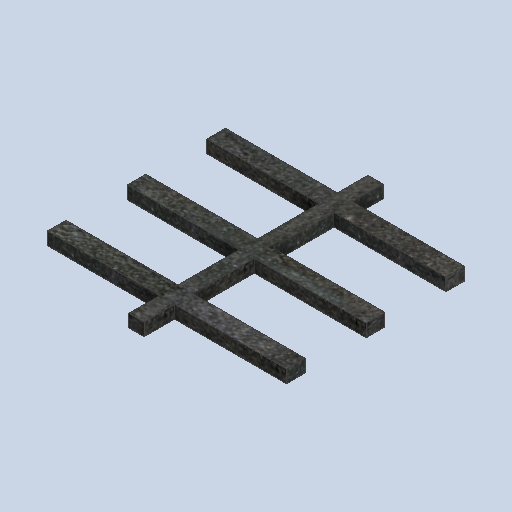
# Autodesk Inventor part: Grid RS3
Saved by Autodesk Inventor 2024.3 (Build 283343000, 343)
## iProperties
Created: 2025-06-18
Part Number: Grid RS3
Material: Steel
Document SubType Name: Modeling
Designer: ajclo
Density: 7.85 g/cm^3
Appearance: Plate
Mass: 98.125 g
Surface Area: 86.4 cm^2
Volume: 12.5 cm^3
Author: ajclo
Autodesk Inventor part; units mm, degrees
ref_plane "YZ Plane" through (0, 0, 0) normal (1, 0, 0) x (0, 1, 0)
ref_plane "XZ Plane" through (0, 0, 0) normal (0, 1, 0) x (-1, 0, 0)
ref_plane "XY Plane" through (0, 0, 0) normal (0, 0, 1) x (1, 0, 0)
sketch "Sketch1" plane through (0, 0, 0) normal (0, 1, 0) x (-1, 0, 0)
  line L0 (-47, 47) -> (47, 47)
  line L1 (47, 47) -> (47, -47)
  line L2 (47, -47) -> (-47, -47)
  line L3 (-47, -47) -> (-47, 47)
  line L4 (-47, 47) -> (47, -47) construction
  line L5 (47, 47) -> (-47, -47) construction
  line L6 (47, -35) -> (3, -35)
  line L7 (3, -35) -> (3, -47)
  line L8 (3, -47) -> (47, -47)
  line L9 (47, -47) -> (47, -35)
  line L10 (47, -3.667) -> (3, -3.667)
  line L11 (3, -3.667) -> (3, -27.667)
  line L12 (3, -27.667) -> (47, -27.667)
  line L13 (47, -27.667) -> (47, -3.667)
  point P0 (0, 0)
  point P1 (25, -47)
  point P2 (25, -35)
  dimension "d0" = 94
  dimension "d1" = 94
  dimension "d2" = 12
  dimension "d3" = 24
  dimension "d4" = 7.333
  dimension "d9" = 3
  dimension "d10" = 0
  constraints: 28 end point, 6 parallel, 4 midpoint, 3 horizontal, 3 perpendicular, 3 point on line
  measures "d0" distance of L0.end L1.end
  measures "d1" distance of L1.end L2.end
  measures "d2" distance of point (25, -47) point (25, -35)
  measures "d3" distance between parallel lines of L12 L10
  measures "d4" distance between parallel lines of L6 L12
  measures "d9" distance from line of point (0, 0) L7
  measures "d10" distance between parallel lines of L7 L11
extrude "Extrusion1" add sketch "Sketch1" along normal blind 5
extrude "Extrusion2" cut sketch "Sketch1" along normal blind 5 contours L1 L12 L11 L10 | L7 L6 L1 L2
mirror "Mirror1" about plane through (0, 0, 0) normal (1, 0, 0) of "Extrusion2"
mirror "Mirror2" about plane through (0, 0, 0) normal (0, 0, 1) of "Extrusion2", "Mirror1"
body "Solid1"
